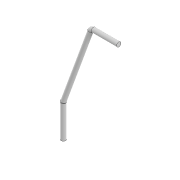
# Autodesk Inventor part: asta
Saved by Autodesk Inventor 2022 (Build 260153000, 153)
## iProperties
Created: 2025-07-13
Part Number: asta
Material: Generic
Document SubType Name: Modeling
Designer: 1234
Density: 1 g/cm^3
Appearance: Default
Author: 1234
Autodesk Inventor part; units mm, degrees
ref_plane "YZ Plane" through (0, 0, 0) normal (1, 0, 0) x (0, 1, 0)
ref_plane "XZ Plane" through (0, 0, 0) normal (0, 1, 0) x (-1, 0, 0)
ref_plane "XY Plane" through (0, 0, 0) normal (0, 0, 1) x (1, 0, 0)
sketch "Sketch1" plane through (0, 0, 0) normal (0, 0, 1) x (1, 0, 0)
  line L0 (0, 0) -> (0, 59.1184)
  line L1 (0.3015, 60.8285) -> (50.1056, 197.664)
  line L2 (54.8041, 200.9539) -> (101.303, 200.9539)
  arc A0 (0.3015, 60.8285) -> (0, 59.1184) centre (5, 59.1184) ccw
  arc A1 (54.8041, 200.9539) -> (50.1056, 197.664) centre (54.8041, 195.9539) ccw
  point P0 (0, 60)
  point P1 (51.303, 200.9539)
  dimension "d0" = 60
  dimension "d1" = 150
  dimension "d2" = 160
  dimension "d3" = 50
  dimension "d4" = 5
  dimension "d5" = 5
  constraints: 6 end point, 4 point on circle, 4 point on line, 4 tangent, 2 centre point, 1 perpendicular, 1 vertical
  measures "d0" distance of L0.start point (0, 60)
  measures "d1" distance of point (0, 60) point (51.303, 200.954)
  measures "d2" angle of L0 L1
  measures "d3" distance of point (51.303, 200.954) L2.end
  measures "d4" radius of A0
  measures "d5" radius of A1
sketch "Sketch2" plane through (0, 0, 0) normal (0, 1, 0) x (-1, 0, 0)
  circle A0 centre (0, 0) radius 4
  dimension "d6" = 8
  constraints: 1 centre point, 1 coincident
  measures "d6" diameter of A0
sweep "Sweep1" add profiles "Sketch2" path "Sketch1" path curves L0 A0 L1 A1 L2
body "Solid1"
